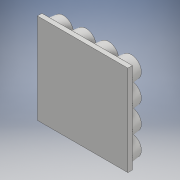
# Autodesk Inventor part: 底座
Saved by Autodesk Inventor 2017 (Build 210142000, 142)
## iProperties
Created: 2021-05-18
Part Number: 底座
Material: Generic
Document SubType Name: Modeling
Designer: user
Density: 1 g/cm^3
Appearance: Default
Author: user
Autodesk Inventor part; units mm, degrees
ref_plane "YZ Plane" through (0, 0, 0) normal (1, 0, 0) x (0, 1, 0)
ref_plane "XZ Plane" through (0, 0, 0) normal (0, 1, 0) x (-1, 0, 0)
ref_plane "XY Plane" through (0, 0, 0) normal (0, 0, 1) x (1, 0, 0)
sketch "Sketch1" plane through (0, 0, 0) normal (0, 1, 0) x (-1, 0, 0)
  line L0 (0, 0) -> (-400, 0)
  line L1 (-400, 0) -> (-400, -400)
  line L2 (-400, -400) -> (0, -400)
  line L3 (0, -400) -> (0, 0)
  dimension "d0" = 400
  dimension "d1" = 400
  constraints: 8 end point, 2 parallel, 1 horizontal, 1 perpendicular
  measures "d0" distance of L1.end L2.end
  measures "d1" distance of L2.end L0.start
extrude "Extrusion1" add sketch "Sketch1" along normal blind 20
ref_plane "Work Plane1" through (0, 0, -50) normal (0, 0, 1) x (1, 0, 0)
sketch "Sketch2" plane through (0, 0, -50) normal (0, 0, 1) x (1, 0, 0)
  line L0 (0, 20) -> (400, 20) projected
  line L1 (0, 20) -> (5.2786, 65)
  arc A0 (5.2786, 65) -> (50, 25) centre (50, 70) ccw
  line L2 (50, 25) -> (50, 20)
  line L3 (0, 20) -> (50, 20)
  line L4 (50, 70) -> (50, 25)
  line L5 (0, 0) -> (0, 20) projected
  dimension "d5" = 45
  dimension "d6" = 50
  dimension "d7" = 5
  dimension "d15" = 40
  constraints: 8 end point, 2 point on circle, 1 centre point, 1 collinear, 1 perpendicular, 1 point on line, 1 vertical
  measures "d5" radius of A0
  measures "d6" distance between parallel lines of L5 L2
  measures "d7" distance of L2.end L2.start
  measures "d15" vertical distance of L2.start L1.end
revolve "Revolution1" add sketch "Sketch2" angle 360 about axis through (50, 25, -50) along (0, -1, 0)
pattern_linear "Rectangular Pattern1" count 4 spacing 100 along (1, 0, 0) count 4 spacing -100 along (0, 0, 1) of "Revolution1"
body "Solid1"
